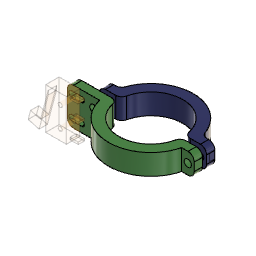
Limitswitch_steering_holder (Autodesk Fusion 360 design; units mm, degrees)
Autodesk Fusion 360 part; units mm, degrees
sketch "Sketch1" plane through (0, 0, 0) normal (0, 0, 1) x (1, 0, 0) in component "limitswitch"
  line L0 (10, 5) -> (-10, 5)
  line L1 (-10, 5) -> (-10, -5)
  line L2 (-10, -5) -> (10, -5)
  line L3 (10, -5) -> (10, 5)
  line L4 (10, 5) -> (-10, -5) construction
  line L5 (-10, 5) -> (10, -5) construction
  circle A0 centre (5, -2) radius 1
  circle A1 centre (-5, -2) radius 1
  dimension "d1" = 20
  dimension "d2" = 10
  dimension "d3" = 2
  dimension "d4" = 2
  dimension "d5" = 3
  dimension "d6" = 5
  dimension "d7" = 5
  constraint horizontal L0
  constraint perpendicular L0 L1
  constraint parallel L0 L2
  constraint parallel L1 L3
  constraint coincident L4 origin
  constraint coincident L5 origin
  constraint horizontal A0.centre A1.centre
  measures "d1" distance of L1.end L2.end
  measures "d2" distance of L0.end L1.end
  measures "d3" diameter of A0
  measures "d4" diameter of A1
  measures "d5" distance of L2 A0.centre
  measures "d6" distance of L3 A0.centre
  measures "d7" distance of L1 A1.centre
extrude "Extrude1" add sketch "Sketch1" along normal blind 6.5 makes body 1 in component "limitswitch"
sketch "Sketch2" plane through (0, -5, 0) normal (0, -1, 0) x (1, 0, 0) in component "limitswitch"
  line L0 (-10, 0) -> (10, 0)
  line L1 (10, 0) -> (10, 6.5)
  line L2 (10, 6.5) -> (-10, 6.5)
  line L3 (-10, 6.5) -> (-10, 0)
  line L4 (-8, 1.75) -> (-9, 1.75)
  line L5 (-9, 1.75) -> (-9, 4.75)
  line L6 (-9, 4.75) -> (-8, 4.75)
  line L7 (-8, 4.75) -> (-8, 1.75)
  line L8 (-8, 1.75) -> (-9, 4.75) construction
  line L9 (-9, 1.75) -> (-8, 4.75) construction
  line L10 (-10, 3.7764) -> (-10, 3.5051)
  line L11 (10, 3.25) -> (-10, 3.25) construction
  line L12 (0.5, 1.75) -> (-0.5, 1.75)
  line L13 (0.5, 1.75) -> (-0.5, 4.75) construction
  line L14 (-0.5, 4.75) -> (0.5, 4.75)
  line L15 (0.5, 4.75) -> (0.5, 1.75)
  line L16 (-0.5, 1.75) -> (0.5, 4.75) construction
  line L17 (-0.5, 1.75) -> (-0.5, 4.75)
  line L18 (9, 1.75) -> (8, 1.75)
  line L19 (9, 1.75) -> (8, 4.75) construction
  line L20 (8, 4.75) -> (9, 4.75)
  line L21 (9, 4.75) -> (9, 1.75)
  line L22 (8, 1.75) -> (9, 4.75) construction
  line L23 (8, 1.75) -> (8, 4.75)
  point P0 (-8.5, 3.25)
  point P1 (0, 3.25)
  point P2 (8.5, 3.25)
  dimension "d10" = 1
  dimension "d11" = 3
  dimension "d12" = 1
  dimension "d13" = 3
  dimension "d14" = 1
  dimension "d15" = 3
  dimension "d16" = 1.5
  dimension "d17" = 1.5
  constraint horizontal L4
  constraint perpendicular L4 L5
  constraint parallel L4 L6
  constraint parallel L5 L7
  constraint coincident L8 P0
  constraint coincident L9 P0
  constraint coincident L3 L10.start
  constraint midpoint L1 L11.start
  constraint midpoint L3 L11.end
  constraint horizontal L12
  constraint perpendicular L12 L17
  constraint parallel L12 L14
  constraint parallel L15 L17
  constraint coincident P1 L13
  constraint coincident P1 L16
  constraint horizontal L18
  constraint perpendicular L18 L23
  constraint parallel L18 L20
  constraint parallel L21 L23
  constraint coincident P2 L19
  constraint coincident P2 L22
  constraint midpoint L11 P1
  constraint coincident L11 P2
  measures "d10" distance of L5.end L6.end
  measures "d11" distance of L4.end L5.end
  measures "d12" distance of L13.end L14.end
  measures "d13" distance of L12.end L13.end
  measures "d14" distance of L19.end L20.end
  measures "d15" distance of L18.end L19.end
  measures "d16" distance of L1 P2
  measures "d17" distance of L3 P0
extrude "Extrude2" add sketch "Sketch2" along normal blind 4 contours L4 L5 L6 L7 | L12 L14 L15 L17 | L18 L20 L21 L23 bodies 1 in component "limitswitch"
ref_plane "WorkPlane1" through (0, 0, 3.25) normal (0, 0, 1) x (1, 0, 0) in component "limitswitch"
sketch "Sketch3" plane through (0, 0, 3.25) normal (0, 0, 1) x (1, 0, 0) in component "limitswitch"
  circle A0 centre (5, -2) radius 1
  circle A1 centre (-5, -2) radius 1
  line L0 (10, -5) -> (10, 5)
  line L1 (10, 5) -> (-10, 5)
  line L2 (-10, 5) -> (-10, -5)
  line L3 (-10, -5) -> (10, -5)
  line L4 (-7, 5) -> (11.3526, 9.9176)
  line L5 (11.3526, 9.9176) -> (10.0585, 14.7472)
  line L6 (10.0585, 14.7472) -> (5.7118, 13.5825)
  line L7 (5.7118, 13.5825) -> (7.0059, 8.7529)
  line L8 (11.3526, 9.9176) -> (11.482, 9.4346)
  line L9 (11.482, 9.4346) -> (-5.0681, 5)
  dimension "d20" = 19
  dimension "d21" = 3
  dimension "d22" = 4.5
  dimension "d23" = 0.5
  dimension "d24" = 15
  dimension "d25" = 5
  constraint coincident L1 L4.start
  constraint perpendicular L4 L5
  constraint coincident L4 L7.end
  constraint perpendicular L4 L7
  constraint perpendicular L4 L8
  constraint coincident L1 L9.end
  constraint parallel L4 L9
  constraint perpendicular L5 L6
  measures "d20" distance of L4.start L4.end
  measures "d21" distance of L2 L4.start
  measures "d22" distance of L5 L7
  measures "d23" distance of L4 L9
  measures "d24" angle of L1 L4
  measures "d25" distance of L4 L6
extrude "Extrude3" add sketch "Sketch3" along normal blind 2 and the other way blind 2 contours L1 L4 L8 L9 | L4 L5 L6 L7 bodies 1 in component "limitswitch"
sketch "Sketch1 (2)" plane through (0, 0, 0) normal (0, 0, 1) x (1, 0, 0) in component "tube_clamp"
  circle A0 centre (0, 0) radius 15
  circle A1 centre (0, 0) radius 15.5
  line L0 (38.2121, 0) -> (-34.1582, 0) construction
  circle A2 centre (0, 0) radius 20.5
  line L1 (26, 0) -> (26, -5)
  line L2 (26, -5) -> (19.8809, -5)
  line L3 (26, -1) -> (20.4756, -1)
  line L4 (-20.4756, -1) -> (-35.4756, -1)
  line L5 (-35.4756, -1) -> (-35.4756, -5)
  line L6 (-35.4756, -5) -> (-19.8809, -5)
  line L7 (-20.4756, -1) -> (-15.4677, -1)
  line L8 (20.4756, -1) -> (15.4677, -1)
  line L9 (20.4756, 1) -> (26, 1)
  line L10 (26, 1) -> (26, 5)
  line L11 (26, 5) -> (19.8809, 5)
  line L12 (-20.4756, 1) -> (-26, 1)
  line L13 (-26, 1) -> (-26, 5)
  line L14 (-26, 5) -> (-19.8809, 5)
  line L15 (20.4756, 1) -> (15.4677, 1)
  line L16 (-20.4756, 1) -> (-15.4677, 1)
  dimension "d30" = 30
  dimension "d32" = 0.5
  dimension "d33" = 5
  dimension "d34" = 26
  dimension "d36" = 1
  dimension "d37" = 4
  dimension "d38" = 1
  dimension "d39" = 4
  dimension "d40" = 15
  dimension "d56" = 26
  dimension "d57" = 1
  dimension "d58" = 4
  dimension "d59" = 26
  dimension "d60" = 1
  dimension "d61" = 4
  constraint coincident A0.centre A1.centre
  constraint horizontal L0
  constraint coincident A0.centre L0
  constraint concentric A1 A2
  constraint coincident L0 L1.start
  constraint perpendicular L0 L1
  constraint coincident A2 L2.end
  constraint perpendicular L1 L2
  constraint coincident L1 L3.start
  constraint coincident A2 L3.end
  constraint perpendicular L1 L3
  constraint coincident A2 L4.start
  constraint parallel L0 L4
  constraint perpendicular L0 L5
  constraint coincident A2 L6.end
  constraint perpendicular L5 L6
  constraint coincident A1 L7.end
  constraint parallel L4 L7
  constraint coincident A1 L8.end
  constraint parallel L3 L8
  constraint coincident A2 L9.start
  constraint parallel L0 L9
  constraint perpendicular L9 L10
  constraint coincident A2 L11.end
  constraint perpendicular L10 L11
  constraint coincident A2 L12.start
  constraint horizontal L12
  constraint perpendicular L12 L13
  constraint coincident A2 L14.end
  constraint perpendicular L13 L14
  constraint coincident A1 L15.end
  constraint parallel L0 L15
  constraint coincident A1 L16.end
  constraint parallel L12 L16
  measures "d30" diameter of A0
  measures "d32" distance of A0 A1
  measures "d33" distance of A1 A2
  measures "d34" distance of A0.centre L1
  measures "d36" distance of L0 L3
  measures "d37" distance of L2 L3
  measures "d38" distance of L0 L4
  measures "d39" distance of L4 L6
  measures "d40" distance of L4.start L5
  measures "d56" distance of A0.centre L10
  measures "d57" distance of L0 L9
  measures "d58" distance of L9 L11
  measures "d59" distance of A0.centre L13
  measures "d60" distance of L0 L12
  measures "d61" distance of L12 L14
extrude "Extrude1'" add sketch "Sketch1 (2)" along normal blind 5 and the other way blind 5 separate body contours A1 A2 L7 L8 | A2 L1 L2 L3 | A2 L4 L5 L6 makes body 2 in component "tube_clamp"
extrude "Extrude4" add sketch "Sketch1 (2)" along normal blind 5 and the other way blind 5 separate body contours A1 A2 L15 L16 | A2 L9 L10 L11 | A2 L12 L13 L14 makes body 3 in component "tube_clamp"
sketch "Sketch2 (2)" plane through (0, -5, 0) normal (0, -1, 0) x (1, 0, 0) in component "tube_clamp"
  line L0 (26, -5) -> (26, 5)
  line L1 (26, 5) -> (19.8809, 5)
  line L2 (19.8809, 5) -> (19.8809, -5)
  line L3 (19.8809, -5) -> (26, -5)
  line L4 (-19.8809, -5) -> (-19.8809, 5)
  line L5 (-19.8809, 5) -> (-35.4756, 5)
  line L6 (-35.4756, 5) -> (-35.4756, -5)
  line L7 (-35.4756, -5) -> (-19.8809, -5)
  circle A0 centre (-22.8809, 0) radius 1.75
  circle A1 centre (22.8809, 0) radius 1.75
  dimension "d45" = 3.5
  dimension "d46" = 3.5
  dimension "d47" = 3
  dimension "d48" = 3
  constraint horizontal A0.centre A1.centre
  constraint horizontal origin A1.centre
  measures "d45" diameter of A0
  measures "d46" diameter of A1
  measures "d47" distance of L2 A1.centre
  measures "d48" distance of L4 A0.centre
extrude "Extrude2'" cut sketch "Sketch2 (2)" against normal blind 19 contours A0 | A1 bodies 2 3 in component "tube_clamp"
sketch "Sketch4" plane through (0, 5, 0) normal (0, 1, 0) x (-1, 0, 0) in component "tube_clamp"
  circle A0 centre (22.8809, 0) radius 1.75
  line L0 (26, -5) -> (26, 5)
  line L1 (26, 5) -> (19.8809, 5)
  line L2 (19.8809, 5) -> (19.8809, -5)
  line L3 (19.8809, -5) -> (26, -5)
  circle A1 centre (-22.8809, 0) radius 1.75
  line L4 (-19.8809, -5) -> (-19.8809, 5)
  line L5 (-19.8809, 5) -> (-26, 5)
  line L6 (-26, 5) -> (-26, -5)
  line L7 (-26, -5) -> (-19.8809, -5)
  line L8 (25.7309, 1.6454) -> (22.8809, 3.2909)
  line L9 (22.8809, 3.2909) -> (20.0309, 1.6454)
  line L10 (20.0309, 1.6454) -> (20.0309, -1.6454)
  line L11 (20.0309, -1.6454) -> (22.8809, -3.2909)
  line L12 (22.8809, -3.2909) -> (25.7309, -1.6454)
  line L13 (25.7309, -1.6454) -> (25.7309, 1.6454)
  line L14 (-22.8809, 3.2909) -> (-25.7309, 1.6454)
  line L15 (-25.7309, 1.6454) -> (-25.7309, -1.6454)
  line L16 (-25.7309, -1.6454) -> (-22.8809, -3.2909)
  line L17 (-22.8809, -3.2909) -> (-20.0309, -1.6454)
  line L18 (-20.0309, -1.6454) -> (-20.0309, 1.6454)
  line L19 (-20.0309, 1.6454) -> (-22.8809, 3.2909)
  point P0 (22.8809, 0)
  point P1 (-22.8809, 0)
  dimension "d66" = 2.85
  dimension "d67" = 2.85
  constraint coincident P0 A0.centre
  constraint coincident P1 A1.centre
  constraint parallel L4 L18
  constraint parallel L2 L13
  measures "d66" distance of P0 L13
  measures "d67" distance of P1 L19
extrude "Extrude5" cut sketch "Sketch4" against normal blind 2.5 contours L8 L9 L10 L11 L12 L13 | L14 L15 L16 L17 L18 L19 bodies 3 in component "tube_clamp"
sketch "Sketch3 (2)" plane through (0, -5, 0) normal (0, -1, 0) x (1, 0, 0) in component "tube_clamp"
  circle A0 centre (-22.8809, 0) radius 1.75
  line L0 (-19.8809, -5) -> (-19.8809, 5)
  line L1 (-19.8809, 5) -> (-35.4756, 5)
  line L2 (-35.4756, 5) -> (-35.4756, -5)
  line L3 (-35.4756, -5) -> (-19.8809, -5)
  line L4 (-35.4756, -5) -> (-35.4756, -13)
  line L5 (-35.4756, -13) -> (-20.4756, -13)
  line L6 (-35.4756, 0) -> (-33.4756, 0) construction
  line L7 (-20.4756, -13) -> (-20.4756, 5)
  dimension "d84" = 18
  dimension "d85" = 15
  constraint coincident L2.end L3.start
  constraint perpendicular L3 L4
  constraint perpendicular L4 L5
  constraint midpoint L2 L6.start
  constraint coincident L1 L7.end
  constraint perpendicular L1 L7
  measures "d84" distance of L1 L5
  measures "d85" distance of L2 L7
extrude "Extrude3'" add sketch "Sketch3 (2)" against normal up to surface (4 mm away) contours L3 L4 L5 L7 | L1 L2 L3 L7 bodies 2 in component "tube_clamp"
sketch "Sketch5" plane through (0, -5, 0) normal (0, -1, 0) x (1, 0, 0) in component "tube_clamp"
  line L0 (-19.8809, -5) -> (-19.8809, 5)
  line L1 (-19.8809, 5) -> (-35.4756, 5)
  line L2 (-35.4756, 5) -> (-35.4756, -13)
  line L3 (-35.4756, -13) -> (-20.4756, -13)
  line L4 (-20.4756, -5) -> (-19.8809, -5)
  circle A0 centre (-31.4756, -9) radius 1
  circle A1 centre (-31.4756, 1) radius 1
  line L5 (-33.4756, -10.25) -> (-28.4756, -10.25)
  arc A2 (-28.4756, -10.25) -> (-28.4756, -7.75) centre (-28.4756, -9) ccw
  line L6 (-28.4756, -7.75) -> (-33.4756, -7.75)
  arc A3 (-33.4756, -7.75) -> (-33.4756, -10.25) centre (-33.4756, -9) ccw
  line L7 (-33.4756, -9) -> (-28.4756, -9) construction
  line L8 (-28.4756, 2.25) -> (-33.4756, 2.25)
  arc A4 (-33.4756, 2.25) -> (-33.4756, -0.25) centre (-33.4756, 1) ccw
  line L9 (-33.4756, -0.25) -> (-28.4756, -0.25)
  arc A5 (-28.4756, -0.25) -> (-28.4756, 2.25) centre (-28.4756, 1) ccw
  line L10 (-28.4756, 1) -> (-33.4756, 1) construction
  line L11 (-20.4756, -13) -> (-20.4756, -5)
  circle A6 centre (-22.8809, 0) radius 1.75
  dimension "d74" = 2.5
  dimension "d75" = 2.5
  dimension "d76" = 2
  dimension "d79" = 2
  dimension "d86" = 7
  constraint tangent L5 A2
  constraint tangent A2 L6
  constraint parallel L5 L6
  constraint tangent L6 A3
  constraint tangent L5 A3
  constraint horizontal L7
  constraint tangent L8 A4
  constraint tangent A4 L9
  constraint parallel L8 L9
  constraint tangent L9 A5
  constraint tangent L8 A5
  constraint horizontal L10
  constraint coincident A1.centre L10
  constraint coincident A0.centre L7
  constraint vertical A2.centre A5.centre
  measures "d74" diameter of A2
  measures "d75" diameter of A4
  measures "d76" distance of L2 A3.centre
  measures "d79" distance of L2 A4.centre
  measures "d86" distance of L2 A2.centre
extrude "Extrude6" cut sketch "Sketch5" against normal blind 5 contours A0 | A1 | L5 A2 L6 A3 | L8 A4 L9 A5 bodies 2 in component "tube_clamp"
fillet "Fillet1" radius 3 16 edges at (-35.4756, -3, -13) (-15.4677, -1, 0) (15.4677, -1, 0) (26, -3, 5) (26, -3, -5) (-35.4756, -3, 5) (-20.4756, -3, -5) (-20.4756, -3, -13) (-26, 3, -5) (-26, 3, 5) (-19.8809, 5, 0) (26, 3, -5) (26, 3, 5) (19.8809, 5, 0) (15.4677, 1, 0) (-15.4677, 1, 0) on bodies 2 3 in component "tube_clamp"
component "limitswitch" placed x (0, 0, -1) y (-1, 0, 0) z (0, 1, 0) at (-33.4756, -12.5, -4)
component "tube_clamp" placed x (1, 0, 0) y (0, 1, 0) z (0, 0, 1) at (0, 0, 0)
equation "d56 = d34"
equation "d57 = d36"
equation "d58 = d37"
equation "d59 = d34"
equation "d60 = d57"
equation "d61 = d37"
named bodies: "Upper_clamp", "Lower_clamp"
